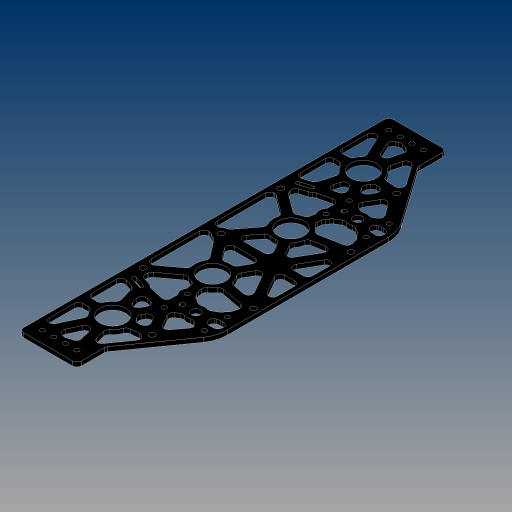
# Autodesk Inventor part: ELEV_027_GEARBOX1
Saved by Autodesk Inventor 2024.3 (Build 283343000, 343)
## iProperties
Created: 2024-12-02
Part Number: ELEV_027_GEARBOX1
Material: Aluminum 6061
Document SubType Name: Modeling
Designer: Kenji
Density: 2.7 g/cm^3
Appearance: Anodized - Black
Mass: 464.349 g
Surface Area: 813.217 cm^2
Volume: 171.981 cm^3
Author: Kenji
Autodesk Inventor part; units mm, degrees
(part 1 of 2)
ref_plane "YZ Plane" through (0, 0, 0) normal (1, 0, 0) x (0, 1, 0)
ref_plane "XZ Plane" through (0, 0, 0) normal (0, 1, 0) x (-1, 0, 0)
ref_plane "XY Plane" through (0, 0, 0) normal (0, 0, 1) x (1, 0, 0)
sketch "Sketch1" plane through (0, 0, 0) normal (0, 1, 0) x (-1, 0, 0)
  line L0 (0, 0) -> (63.5, 0) construction
  line L1 (63.5, 0) -> (63.5, -25.4) construction
  line L2 (63.5, -25.4) -> (0, -25.4) construction
  line L3 (0, -25.4) -> (0, 0) construction
  line L4 (0, -381) -> (63.5, -381) construction
  line L5 (63.5, -381) -> (63.5, -406.4) construction
  line L6 (63.5, -406.4) -> (0, -406.4) construction
  line L7 (0, -406.4) -> (0, -381) construction
  circle A0 centre (26.0346, -341.0966) radius 22.733 construction
  circle A1 centre (26.0346, -65.3034) radius 22.733 construction
  line L8 (26.0346, -65.3034) -> (26.0346, -341.0966) construction
  line L9 (63.5, -203.2) -> (-50.8, -203.2) construction
  circle A2 centre (26.0346, -65.3034) radius 14.2875
  circle A3 centre (26.0346, -341.0966) radius 14.2875
  circle A4 centre (26.0346, -65.3034) radius 27.2288 construction
  circle A5 centre (26.0346, -341.0966) radius 27.2288 construction
  circle A6 centre (692.1496, -341.0966) radius 22.733 construction
  circle A7 centre (692.1496, -341.0966) radius 27.2288 construction
  line L10 (-50.8, 0) -> (-50.8, -406.4) construction
  circle A8 centre (-16.5354, -292.1) radius 31.7246 construction
  circle A9 centre (-16.5354, -114.3) radius 31.7246 construction
  circle A10 centre (-16.5354, -292.1) radius 10.16 construction
  circle A11 centre (-16.5354, -114.3) radius 10.16 construction
  circle A12 centre (-16.5354, -292.1) radius 5
  circle A13 centre (-16.5354, -114.3) radius 5
  line L11 (692.1496, -363.8296) -> (26.0346, -363.8296) construction
  line L12 (-48.26, -114.3) -> (-50.8, -114.3) construction
  line L13 (63.5, -25.4) -> (63.5, -381) construction
  line L14 (-48.26, -292.1) -> (-50.8, -292.1) construction
  circle A14 centre (10.9389, -160.02) radius 43.18 construction
  circle A15 centre (10.9389, -160.02) radius 45.72 construction
  circle A16 centre (10.9389, -246.38) radius 43.18 construction
  line L15 (10.9389, -160.02) -> (10.9389, -246.38) construction
  circle A17 centre (10.9389, -160.02) radius 14.2875
  circle A18 centre (10.9389, -246.38) radius 14.2875
  circle A19 centre (10.9389, -246.38) radius 45.72 construction
  line L16 (10.9389, -203.2) -> (63.5, -203.2) construction
  circle A20 centre (10.9389, -160.02) radius 14.3256 construction
  circle A21 centre (26.0346, -65.3034) radius 28.6512 construction
  circle A22 centre (26.0346, -341.0966) radius 28.6512 construction
  circle A23 centre (10.9389, -246.38) radius 14.3256 construction
  line L17 (53.3378, -73.9883) -> (24.5905, -164.3625) construction
  line L18 (-2.6157, -65.0706) -> (-3.3862, -159.9036) construction
  line L19 (53.3378, -332.4117) -> (24.5905, -242.0375) construction
  line L20 (-3.3862, -246.4964) -> (-2.6157, -341.3294) construction
  circle A24 centre (12.7, -12.7) radius 2.54
  line L21 (63.5, -12.7) -> (0, -12.7) construction
  circle A25 centre (25.4, -12.7) radius 2.54
  circle A26 centre (38.1, -12.7) radius 2.54
  circle A27 centre (50.8, -12.7) radius 2.54
  circle A28 centre (12.7, -393.7) radius 2.54
  circle A29 centre (25.4, -393.7) radius 2.54
  circle A30 centre (38.1, -393.7) radius 2.54
  circle A31 centre (50.8, -393.7) radius 2.54
  line L22 (63.5, -401.6375) -> (63.5, -4.7625)
  line L23 (58.7375, 0) -> (4.7625, 0)
  line L24 (0, -4.7625) -> (0, -25.4)
  circle A32 centre (-16.5354, -114.3) radius 34.2646 construction
  line L25 (0, 0) -> (-50.8, 0) construction
  line L26 (-50.8, 0) -> (-50.8, -25.4) construction
  line L27 (-50.8, -25.4) -> (0, -25.4) construction
  line L28 (0, -25.4) -> (0, 0) construction
  line L29 (0, -25.4) -> (0, -30.2327)
  line L30 (-0.8777, -32.9877) -> (-44.4852, -94.479)
  arc A33 (-0.8777, -32.9877) -> (0, -30.2327) centre (-4.7625, -30.2327) ccw
  circle A34 centre (-16.5354, -292.1) radius 34.2646 construction
  line L31 (-50.8, -114.3) -> (-50.8, -292.1)
  line L32 (58.7375, -406.4) -> (4.7625, -406.4)
  line L33 (0, -381) -> (0, -401.6375)
  line L34 (0, -381) -> (0, -376.1673)
  line L35 (-0.8777, -373.4123) -> (-44.4852, -311.921)
  arc A35 (0, -376.1673) -> (-0.8777, -373.4123) centre (-4.7625, -376.1673) ccw
  arc A36 (-44.4852, -94.479) -> (-50.8, -114.3) centre (-16.5354, -114.3) ccw
  arc A37 (-50.8, -292.1) -> (-44.4852, -311.921) centre (-16.5354, -292.1) ccw
  arc A38 (4.7625, 0) -> (0, -4.7625) centre (4.7625, -4.7625) ccw
  arc A39 (63.5, -4.7625) -> (58.7375, 0) centre (58.7375, -4.7625) ccw
  arc A40 (58.7375, -406.4) -> (63.5, -401.6375) centre (58.7375, -401.6375) ccw
  arc A41 (0, -401.6375) -> (4.7625, -406.4) centre (4.7625, -401.6375) ccw
  circle A42 centre (50.2604, -112.9905) radius 6.35 construction
  circle A43 centre (50.2604, -112.9905) radius 3.175 construction
  line L36 (50.2604, -112.9905) -> (41.7887, -110.2957) construction
  circle A44 centre (50.2604, -112.9905) radius 1.9844 construction
  line L37 (50.2604, -112.9905) -> (38.1579, -109.1408) construction
  circle A45 centre (38.1579, -109.1408) radius 1.9844 construction
  line L38 (50.8619, -111.0995) -> (38.7594, -107.2498)
  line L39 (49.6589, -114.8815) -> (37.5564, -111.0318)
  arc A46 (49.6589, -114.8815) -> (50.8619, -111.0995) centre (50.2604, -112.9905) ccw
  arc A47 (38.7594, -107.2498) -> (37.5564, -111.0318) centre (38.1579, -109.1408) ccw
  line L40 (50.8619, -295.3005) -> (38.7594, -299.1502)
  line L41 (49.6589, -291.5185) -> (37.5564, -295.3682)
  arc A48 (50.8619, -295.3005) -> (49.6589, -291.5185) centre (50.2604, -293.4095) ccw
  arc A49 (37.5564, -295.3682) -> (38.7594, -299.1502) centre (38.1579, -297.2592) ccw
  circle A50 centre (44.3715, -203.2) radius 6.35 construction
  circle A51 centre (54.8316, -127.5288) radius 6.35 construction
  circle A52 centre (-13.904, -68.6812) radius 6.35 construction
  circle A53 centre (-44.45, -149.4985) radius 6.35 construction
  line L42 (-33.9779, -151.4878) -> (-38.2116, -150.6836) construction
  line L43 (-37.8265, -141.1468) -> (-40.5043, -144.5232) construction
  circle A54 centre (-44.45, -149.4985) radius 3.2512
  line L44 (-2.5147, -67.718) -> (-7.5766, -68.1461) construction
  line L45 (-14.2697, -75.0207) -> (-14.5622, -80.0923) construction
  circle A55 centre (-13.904, -68.6812) radius 3.2512
  line L46 (52.927, -121.4712) -> (52.1651, -119.0481) construction
  line L47 (49.7278, -131.3068) -> (47.6863, -132.8181) construction
  line L48 (40.484, -198.1791) -> (38.929, -196.1707) construction
  line L49 (40.484, -208.2209) -> (38.929, -210.2293) construction
  circle A56 centre (54.8316, -127.5288) radius 3.2512
  circle A57 centre (44.3715, -203.2) radius 3.2512
  circle A58 centre (54.8316, -278.8712) radius 6.35 construction
  circle A59 centre (-13.904, -337.7188) radius 6.35 construction
  circle A60 centre (-44.45, -256.9015) radius 6.35 construction
  circle A61 centre (-44.45, -256.9015) radius 3.2512
  circle A62 centre (-13.904, -337.7188) radius 3.2512
  circle A63 centre (54.8316, -278.8712) radius 3.2512
  circle A64 centre (-16.5354, -114.3) radius 25.4 construction
  circle A65 centre (-16.5354, -88.9) radius 2.54 construction
  circle A66 centre (-29.2354, -92.303) radius 2.54 construction
  circle A67 centre (-38.5324, -101.6) radius 2.54
  circle A68 centre (-41.9354, -114.3) radius 2.54 construction
  circle A69 centre (-38.5324, -127) radius 2.54
  circle A70 centre (-29.2354, -136.297) radius 2.54 construction
  circle A71 centre (-16.5354, -139.7) radius 2.54 construction
  circle A72 centre (-3.8354, -136.297) radius 2.54 construction
  circle A73 centre (5.4616, -127) radius 2.54
  circle A74 centre (8.8646, -114.3) radius 2.54 construction
  circle A75 centre (5.4616, -101.6) radius 2.54
  circle A76 centre (-3.8354, -92.303) radius 2.54 construction
  circle A77 centre (-16.5354, -317.5) radius 2.54 construction
  circle A78 centre (-38.5324, -304.8) radius 2.54
  circle A79 centre (-38.5324, -279.4) radius 2.54
  circle A80 centre (-16.5354, -266.7) radius 2.54 construction
  circle A81 centre (5.4616, -279.4) radius 2.54
  circle A82 centre (5.4616, -304.8) radius 2.54
  circle A83 centre (50.2604, -112.9905) radius 8.89 construction
  line L50 (26.0346, -341.0966) -> (54.8316, -278.8712) construction
  line L51 (26.0346, -341.0966) -> (-13.904, -337.7188) construction
  line L52 (26.0346, -341.0966) -> (12.7, -393.7) construction
  point P0 (0, -31.75)
  point P1 (0, -374.65)
  dimension "d18" = 63.4492
  dimension "d26" = 63.4492
  dimension "d77" = 12.7
  dimension "d93" = 50.8
  dimension "d0" = 25.4
  dimension "d1" = 63.5
  dimension "d2" = 406.4
  dimension "d3" = 45.466
  dimension "d4" = 65.3034
  dimension "d5" = 203.2
  dimension "d6" = 28.575
  dimension "d7" = 54.4576
  dimension "d13" = 692.1496
  dimension "d14" = 50.8
  dimension "d19" = 20.32
  dimension "d33" = 10
  dimension "d34" = 666.115
  dimension "d35" = 2.54
  dimension "d48" = 2.54
  dimension "d49" = 86.36
  dimension "d50" = 28.575
  dimension "d51" = 28.575
  dimension "d52" = 43.18
  dimension "d53" = 177.8
  dimension "d54" = 177.8
  dimension "d56" = 57.3024
  dimension "d58" = 28.6512
  dimension "d59" = 12.7
  dimension "d60" = 5.08
  dimension "d63" = 12.7
  dimension "d68" = 2.54
  dimension "d69" = 25.4
  dimension "d70" = 6.35
  dimension "d71" = 4.7625
  dimension "d72" = 2.54
  dimension "d73" = 6.35
  dimension "d74" = 4.7625
  dimension "d75" = 4.7625
  dimension "d76" = 4.7625
  dimension "d78" = 6.35
  dimension "d81" = 38.1
  dimension "d83" = 3.9688
  dimension "d84" = 12.7
  dimension "d85" = 12.7
  dimension "d86" = 6.5024
  dimension "d87" = 5.08
  dimension "d88" = 6.5024
  dimension "d89" = 2.54
  dimension "d90" = 6.5024
  dimension "d91" = 2.54
  dimension "d92" = 6.5024
  dimension "d94" = 5.08
  dimension "d97" = 360
  dimension "d102" = 2.54
  dimension "d207" = 68.5658
  dimension "d209" = 40.0812
  dimension "d211" = 54.2672
  dimension "d215" = 24.834
  dimension "d216" = 85.166
  dimension "d217" = 80.61
  constraints: 106 end point, 77 centre point, 54 point on circle, 40 point on line, 32 tangent, 26 coincident, 22 symmetric about line, 15 equal radius, 7 horizontal, 7 parallel, 7 perpendicular, 6 collinear, 6 equal length, 6 midpoint, 6 vertical, 4 vertical alignment, 3 concentric, 3 horizontal alignment, 68 other
  measures "d0" distance between parallel lines of L0 L2
  measures "d1" distance of L0.start L0.end
  measures "d2" distance between parallel lines of L6 L0
  measures "d3" diameter of A1
  measures "d4" distance from line of L6 L8.end
  measures "d5" distance between parallel lines of L6 L9
  measures "d6" diameter of A2
  measures "d7" diameter of A4
  measures "d13" distance from line of L7 point (692.15, -341.097)
  measures "d14" distance between parallel lines of L10 L7
  measures "d19" diameter of A10
  measures "d33" diameter of A13
  measures "d34" distance of L11.start L11.end
  measures "d35" distance of L12.start L12.end
  measures "d48" radial gap between concentric circles of A14 A15
  measures "d49" diameter of A14
  measures "d50" diameter of A17
  measures "d51" diameter of A18
  measures "d52" distance from line of L15.start L16
  measures "d53" distance between parallel lines of L4 L16
  measures "d54" distance of A34.centre A32.centre
  measures "d56" diameter of A21
  measures "d58" diameter of A20
  measures "d59" distance from line of L3 A24.centre
  measures "d60" diameter of A24
  measures "d63" distance of A24.centre A25.centre
  measures "d69" distance between parallel lines of L25 L27
  measures "d70" distance of L27.end point (0, -31.75)
  measures "d71" radius of A33
  measures "d73" distance of L4.start point (0, -374.65)
  measures "d74" radius of A35
  measures "d75" radius of A38
  measures "d76" radius of A39
  measures "d78" diameter of A43
  measures "d81" distance of L36.end L17.start
  measures "d83" diameter of A44
  measures "d84" distance of L37.start L37.end
  measures "d85" diameter of A50
  measures "d86" diameter of A54
  measures "d87" distance of L44.start L44.end
  measures "d88" diameter of A55
  measures "d89" distance of L46.start L46.end
  measures "d90" diameter of A56
  measures "d91" distance of L48.start L48.end
  measures "d92" diameter of A57
  measures "d94" diameter of A65
  measures "d207" distance of L50.start L50.end
  measures "d209" distance of L50.start A59.centre
  measures "d211" distance of L50.start L52.end
  measures "d215" angle of L8 L50
  measures "d216" angle of L51 L8
  measures "d217" angle of L51 L52
extrude "Extrusion1" add sketch "Sketch1" along normal blind 4.7625
sketch "Sketch2" plane through (0, 4.7625, 0) normal (0, 1, 0) x (1, 0, 0)
  line L0 (-63.5, 401.6375) -> (-63.5, 4.7625) construction
  arc A0 (-63.5, 4.7625) -> (-58.7375, 0) centre (-58.7375, 4.7625) ccw construction
  line L1 (-58.7375, 0) -> (-4.7625, 0) construction
  arc A1 (-4.7625, 0) -> (0, 4.7625) centre (-4.7625, 4.7625) ccw construction
  line L2 (0, 4.7625) -> (0, 30.2327) construction
  arc A2 (0.8777, 32.9877) -> (0, 30.2327) centre (4.7625, 30.2327) ccw construction
  line L3 (0.8777, 32.9877) -> (44.4852, 94.479) construction
  arc A3 (44.4852, 94.479) -> (50.8, 114.3) centre (16.5354, 114.3) ccw construction
  line L4 (50.8, 114.3) -> (50.8, 292.1) construction
  arc A4 (50.8, 292.1) -> (44.4852, 311.921) centre (16.5354, 292.1) ccw construction
  line L5 (44.4852, 311.921) -> (0.8777, 373.4123) construction
  arc A5 (0, 376.1673) -> (0.8777, 373.4123) centre (4.7625, 376.1673) ccw construction
  line L6 (0, 376.1673) -> (0, 401.6375) construction
  arc A6 (0, 401.6375) -> (-4.7625, 406.4) centre (-4.7625, 401.6375) ccw construction
  line L7 (-4.7625, 406.4) -> (-58.7375, 406.4) construction
  arc A7 (-58.7375, 406.4) -> (-63.5, 401.6375) centre (-58.7375, 401.6375) ccw construction
  circle A8 centre (38.5324, 304.8) radius 2.54 construction
  circle A9 centre (-5.4616, 304.8) radius 2.54 construction
  circle A10 centre (-5.4616, 127) radius 2.54 construction
  circle A11 centre (38.5324, 127) radius 2.54 construction
  circle A12 centre (44.45, 256.9015) radius 3.2512 construction
  circle A13 centre (-44.3715, 203.2) radius 3.2512 construction
  circle A14 centre (44.45, 149.4985) radius 3.2512 construction
  circle A15 centre (-25.4, 393.7) radius 2.54 construction
  circle A16 centre (-50.8, 393.7) radius 2.54 construction
  circle A17 centre (-38.1, 12.7) radius 2.54 construction
  circle A18 centre (-26.0346, 65.3034) radius 14.2875 construction
  circle A19 centre (-26.0346, 341.0966) radius 14.2875 construction
  circle A20 centre (16.5354, 292.1) radius 5 construction
  circle A21 centre (16.5354, 114.3) radius 5 construction
  circle A22 centre (-10.9389, 160.02) radius 14.2875 construction
  circle A23 centre (-10.9389, 246.38) radius 14.2875 construction
  circle A24 centre (-12.7, 12.7) radius 2.54 construction
  circle A25 centre (-25.4, 12.7) radius 2.54 construction
  circle A26 centre (-50.8, 12.7) radius 2.54 construction
  circle A27 centre (-38.1, 393.7) radius 2.54 construction
  circle A28 centre (-12.7, 393.7) radius 2.54 construction
  circle A29 centre (-54.8316, 127.5288) radius 3.2512 construction
  circle A30 centre (-54.8316, 278.8712) radius 3.2512 construction
  circle A31 centre (38.5324, 101.6) radius 2.54 construction
  circle A32 centre (-5.4616, 101.6) radius 2.54 construction
  circle A33 centre (-5.4616, 279.4) radius 2.54 construction
  circle A34 centre (38.5324, 279.4) radius 2.54 construction
  circle A35 centre (13.904, 337.7188) radius 3.2512 construction
  circle A36 centre (13.904, 68.6812) radius 3.2512 construction
  line L8 (-50.8619, 295.3005) -> (-38.7594, 299.1502) construction
  arc A37 (-37.5564, 295.3682) -> (-38.7594, 299.1502) centre (-38.1579, 297.2592) ccw construction
  line L9 (-37.5564, 295.3682) -> (-49.6589, 291.5185) construction
  arc A38 (-50.8619, 295.3005) -> (-49.6589, 291.5185) centre (-50.2604, 293.4095) ccw construction
  line L10 (-49.6589, 114.8815) -> (-37.5564, 111.0318) construction
  arc A39 (-38.7594, 107.2498) -> (-37.5564, 111.0318) centre (-38.1579, 109.1408) ccw construction
  line L11 (-38.7594, 107.2498) -> (-50.8619, 111.0995) construction
  arc A40 (-49.6589, 114.8815) -> (-50.8619, 111.0995) centre (-50.2604, 112.9905) ccw construction
  line L12 (-58.7375, 4.7625) -> (-58.7375, 401.6375) construction
  line L13 (-58.7375, 401.6375) -> (-4.7625, 401.6375) construction
  line L14 (-4.7625, 401.6375) -> (-4.7625, 376.1673) construction
  arc A41 (-4.7625, 376.1673) -> (-3.0071, 370.6574) centre (4.7625, 376.1673) ccw construction
  line L15 (-3.0071, 370.6574) -> (40.6004, 309.166) construction
  arc A42 (46.0375, 292.1) -> (40.6004, 309.166) centre (16.5354, 292.1) ccw construction
  line L16 (46.0375, 292.1) -> (46.0375, 203.2) construction
  circle A43 centre (-50.8, 393.7) radius 7.3025 construction
  circle A44 centre (-38.1, 393.7) radius 7.3025 construction
  circle A45 centre (-25.4, 393.7) radius 7.3025 construction
  circle A46 centre (-12.7, 393.7) radius 7.3025 construction
  circle A47 centre (-26.0346, 341.0966) radius 19.05 construction
  circle A48 centre (13.904, 337.7188) radius 8.0137 construction
  circle A49 centre (-5.4616, 304.8) radius 7.3025 construction
  circle A50 centre (-5.4616, 279.4) radius 7.3025 construction
  circle A51 centre (-10.9389, 246.38) radius 19.05 construction
  line L17 (-48.2152, 286.98) -> (-36.1128, 290.8297) construction
  arc A52 (-36.1128, 290.8297) -> (-40.2031, 303.6886) centre (-38.1579, 297.2592) ccw construction
  line L18 (-40.2031, 303.6886) -> (-52.3056, 299.8389) construction
  arc A53 (-52.3056, 299.8389) -> (-48.2152, 286.98) centre (-50.2604, 293.4095) ccw construction
  circle A54 centre (-54.8316, 278.8712) radius 8.0137 construction
  circle A55 centre (-44.3715, 203.2) radius 8.0137 construction
  circle A56 centre (16.5354, 292.1) radius 9.7625 construction
  circle A57 centre (38.5324, 279.4) radius 7.3025 construction
  circle A58 centre (44.45, 256.9015) radius 8.0137 construction
  circle A59 centre (38.5324, 304.8) radius 7.3025 construction
  line L19 (-58.7375, 203.2) -> (46.0375, 203.2) construction
  line L20 (-39.4655, 209.5364) -> (-22.6014, 231.3172) construction
  line L21 (-26.2503, 257.7141) -> (-48.3906, 274.1033) construction
  line L22 (-31.5836, 298.7754) -> (-12.5774, 303.1589) construction
  line L23 (-7.8215, 265.1732) -> (-6.6566, 272.1959) construction
  line L24 (7.7764, 249.9351) -> (36.5771, 255.406) construction
  line L25 (42.4116, 264.6516) -> (40.39, 272.3377) construction
  line L26 (24.99, 287.2188) -> (32.2083, 283.0513) construction
  line L27 (0.8625, 283.0513) -> (8.0808, 287.2188) construction
  line L28 (0.8625, 301.1488) -> (8.0808, 296.9813) construction
  line L29 (24.99, 296.9813) -> (32.2083, 301.1488) construction
  line L30 (18.7047, 331.3021) -> (34.1578, 310.6472) construction
  line L31 (-9.0625, 311.153) -> (-16.641, 324.5236) construction
  line L32 (-1.7589, 311.0941) -> (9.8407, 330.8116) construction
  line L33 (-7.0523, 339.4912) -> (5.9188, 338.3941) construction
  line L34 (-21.3536, 359.5625) -> (-14.4944, 386.6214) construction
  line L35 (-34.1489, 358.332) -> (-47.6895, 387.0931) construction
  line L36 (-36.3596, 303.762) -> (-31.1123, 322.7358) construction
  line L37 (-54.8316, 278.8712) -> (-50.2604, 293.4095) construction
  line L38 (-5.4616, 286.7025) -> (-5.4616, 297.4975) construction
  line L39 (40.4726, 249.9445) -> (13.7479, 203.2) construction
  line L40 (-1.4838, 229.842) -> (13.7479, 203.2) construction
  line L41 (-45.0846, 341.0966) -> (-58.7375, 341.0966) construction
  line L42 (-47.8591, 345.8591) -> (-53.975, 345.8591)
  line L43 (-50.8, 393.7) -> (-58.7375, 393.7) construction
  line L44 (-39.6396, 358.8137) -> (-49.6661, 380.1107)
  arc A60 (-40.3657, 353.6474) -> (-43.4942, 348.7166) centre (-26.0346, 341.0966) ccw
  line L45 (-58.7375, 350.6216) -> (-58.7375, 378.0821)
  arc A61 (-47.8591, 345.8591) -> (-43.4942, 348.7166) centre (-47.8591, 350.6216) ccw
  arc A62 (-40.3657, 353.6474) -> (-39.6396, 358.8137) centre (-43.9484, 356.7851) ccw
  arc A63 (-58.7375, 350.6216) -> (-53.975, 345.8591) centre (-53.975, 350.6216) ccw
  arc A64 (-49.6661, 380.1107) -> (-58.7375, 378.0821) centre (-53.975, 378.0821) ccw
  line L46 (-33.046, 367.1702) -> (-39.1165, 380.0643)
  line L47 (-24.1207, 368.0285) -> (-20.9678, 380.4662)
  arc A65 (-36.1072, 386.6747) -> (-34.2566, 387.4908) centre (-38.1, 393.7) ccw
  arc A66 (-29.2434, 387.4908) -> (-25.5116, 386.3984) centre (-25.4, 393.7) ccw
  arc A67 (-33.046, 367.1702) -> (-24.1207, 368.0285) centre (-28.7371, 369.1988) ccw
  arc A68 (-36.1072, 386.6747) -> (-39.1165, 380.0643) centre (-34.8076, 382.0929) ccw
  arc A69 (-29.2434, 387.4908) -> (-34.2566, 387.4908) centre (-31.75, 383.4413) ccw
  circle A70 centre (-25.5843, 381.6364) radius 4.7625 construction
  arc A71 (-20.9678, 380.4662) -> (-25.5116, 386.3984) centre (-25.5843, 381.6364) ccw
  line L48 (-16.0554, 361.0817) -> (-13.3658, 371.6918)
  line L49 (-3.8863, 344.0029) -> (5.8207, 343.1819)
  line L50 (-12.7, 393.7) -> (-4.7625, 393.7) construction
  line L51 (10.8092, 351.1749) -> (-4.8645, 373.2765)
  arc A72 (-7.9949, 347.2181) -> (-14.358, 356.1485) centre (-26.0346, 341.0966) ccw
  arc A73 (9.5261, 344.431) -> (9.0856, 344.1221) centre (13.904, 337.7188) ccw
  arc A74 (-16.0554, 361.0817) -> (-14.358, 356.1485) centre (-11.4389, 359.9115) ccw
  arc A75 (-7.9949, 347.2181) -> (-3.8863, 344.0029) centre (-3.485, 348.7485) ccw
  arc A76 (5.8207, 343.1819) -> (9.0856, 344.1221) centre (6.222, 347.9275) ccw
  arc A77 (9.5261, 344.431) -> (10.8092, 351.1749) centre (6.9244, 348.42) ccw
  circle A78 centre (-8.7493, 370.5216) radius 4.7625 construction
  arc A79 (-4.8645, 373.2765) -> (-13.3658, 371.6918) centre (-8.7493, 370.5216) ccw
  line L52 (-4.6891, 334.5118) -> (-1.5787, 334.2487)
  line L53 (-1.2033, 321.431) -> (2.1248, 327.0883)
  line L54 (-9.4515, 321.4974) -> (-11.1297, 324.4583)
  arc A80 (-10.796, 329.6646) -> (-9.2793, 332.0323) centre (-26.0346, 341.0966) ccw
  arc A81 (-10.796, 329.6646) -> (-11.1297, 324.4583) centre (-6.9864, 326.8067) ccw
  arc A82 (-4.6891, 334.5118) -> (-9.2793, 332.0323) centre (-5.0904, 329.7662) ccw
  arc A83 (2.1248, 327.0883) -> (-1.5787, 334.2487) centre (-1.9801, 329.5032) ccw
  arc A84 (-9.4515, 321.4974) -> (-1.2033, 321.431) centre (-5.3082, 323.8458) ccw
  line L55 (-47.8591, 336.3341) -> (-53.975, 336.3341)
  line L56 (-40.7412, 305.7855) -> (-36.442, 321.3311)
  line L57 (-56.6898, 291.3643) -> (-58.7375, 290.713) construction
  line L58 (-58.7375, 304.3029) -> (-58.7375, 331.5716)
  arc A85 (-43.4942, 333.4766) -> (-38.0327, 326.2997) centre (-26.0346, 341.0966) ccw
  arc A86 (-52.3056, 299.8389) -> (-52.4379, 299.7953) centre (-50.2604, 293.4095) ccw
  line L59 (-52.3056, 299.8389) -> (-43.8878, 302.5165)
  arc A87 (-43.8878, 302.5165) -> (-40.7412, 305.7855) centre (-45.3314, 307.055) ccw
  arc A88 (-36.442, 321.3311) -> (-38.0327, 326.2997) centre (-41.0322, 322.6005) ccw
  arc A89 (-43.4942, 333.4766) -> (-47.8591, 336.3341) centre (-47.8591, 331.5716) ccw
  arc A90 (-53.975, 336.3341) -> (-58.7375, 331.5716) centre (-53.975, 331.5716) ccw
  circle A91 centre (-53.975, 304.3029) radius 4.7625 construction
  arc A92 (-58.7375, 304.3029) -> (-52.4379, 299.7953) centre (-53.975, 304.3029) ccw
  line L60 (-29.3048, 311.4041) -> (-27.5732, 317.6656)
  line L61 (-23.6444, 305.494) -> (-18.9742, 306.5711)
  line L62 (-15.9012, 313.5602) -> (-18.8398, 318.7446)
  arc A93 (-26.3609, 322.0494) -> (-21.0825, 322.7015) centre (-26.0346, 341.0966) ccw
  arc A94 (-29.3048, 311.4041) -> (-23.6444, 305.494) centre (-24.7146, 310.1347) ccw
  arc A95 (-18.9742, 306.5711) -> (-15.9012, 313.5602) centre (-20.0445, 311.2118) ccw
  arc A96 (-18.8398, 318.7446) -> (-27.5732, 317.6656) centre (-22.983, 316.3962) ccw
  line L63 (-25.6468, 263.1927) -> (-45.1542, 277.6329)
  line L64 (-30.7922, 294.0704) -> (-16.0569, 297.4689)
  line L65 (-10.2241, 286.8053) -> (-10.2241, 292.8282)
  line L66 (-12.0658, 268.6897) -> (-11.3718, 272.8739)
  arc A97 (-15.5991, 264.8512) -> (-20.4384, 262.8925) centre (-10.9389, 246.38) ccw
  arc A98 (-11.2268, 283.8822) -> (-11.8825, 275.9217) centre (-5.4616, 279.4) ccw
  arc A99 (-46.9843, 280.4955) -> (-47.3989, 281.8669) centre (-54.8316, 278.8712) ccw
  arc A100 (-36.1128, 290.8297) -> (-33.2127, 292.6695) centre (-38.1579, 297.2592) ccw
  line L67 (-44.4253, 288.1856) -> (-36.1128, 290.8297)
  arc A101 (-25.6468, 263.1927) -> (-20.4384, 262.8925) centre (-22.8133, 267.0206) ccw
  arc A102 (-15.5991, 264.8512) -> (-12.0658, 268.6897) centre (-16.7641, 269.469) ccw
  arc A103 (-11.3718, 272.8739) -> (-11.8825, 275.9217) centre (-16.0701, 273.6532) ccw
  arc A104 (-11.2268, 283.8822) -> (-10.2241, 286.8053) centre (-14.9866, 286.8053) ccw
  arc A105 (-10.2241, 292.8282) -> (-16.0569, 297.4689) centre (-14.9866, 292.8282) ccw
  arc A106 (-30.7922, 294.0704) -> (-33.2127, 292.6695) centre (-29.7219, 289.4297) ccw
  arc A107 (-46.9843, 280.4955) -> (-45.1542, 277.6329) centre (-42.3206, 281.4608) ccw
  circle A108 centre (-42.9817, 283.6472) radius 4.7625 construction
  arc A109 (-44.4253, 288.1856) -> (-47.3989, 281.8669) centre (-42.9817, 283.6472) ccw
  line L68 (3.5125, 310.6622) -> (10.7493, 322.9636)
  line L69 (5.2361, 304.1229) -> (9.4199, 301.7074)
  line L70 (23.6509, 301.7074) -> (26.8599, 303.5601)
  line L71 (18.6675, 323.4018) -> (28.292, 310.5375)
  arc A110 (19.7173, 301.3294) -> (13.3535, 301.3294) centre (16.5354, 292.1) ccw
  arc A111 (1.7137, 306.1565) -> (1.4502, 307.1565) centre (-5.4616, 304.8) ccw
  arc A112 (3.5125, 310.6622) -> (5.2361, 304.1229) centre (7.6174, 308.2474) ccw
  arc A113 (9.4199, 301.7074) -> (13.3535, 301.3294) centre (11.8012, 305.8318) ccw
  arc A114 (19.7173, 301.3294) -> (23.6509, 301.7074) centre (21.2696, 305.8318) ccw
  arc A115 (26.8599, 303.5601) -> (28.292, 310.5375) centre (24.4786, 307.6845) ccw
  arc A116 (18.6675, 323.4018) -> (10.7493, 322.9636) centre (14.8541, 320.5488) ccw
  line L72 (38.5324, 279.4) -> (46.0375, 279.4) construction
  line L73 (33.2042, 287.9756) -> (34.5005, 287.2271)
  line L74 (33.2042, 296.2244) -> (34.5005, 296.9729)
  arc A117 (33.2042, 296.2244) -> (33.2042, 287.9756) centre (35.5854, 292.1) ccw
  arc A118 (40.1924, 286.5113) -> (37.5333, 286.6338) centre (38.5324, 279.4) ccw
  line L75 (46.0375, 291.1492) -> (46.0375, 292.1)
  arc A119 (37.5333, 297.5662) -> (39.6449, 297.5827) centre (38.5324, 304.8) ccw
  arc A120 (34.5005, 287.2271) -> (37.5333, 286.6338) centre (36.8818, 291.3515) ccw
  arc A121 (37.5333, 297.5662) -> (34.5005, 296.9729) centre (36.8818, 292.8485) ccw
  circle A122 centre (41.275, 291.1492) radius 4.7625 construction
  arc A123 (46.0375, 292.1) -> (39.6449, 297.5827) centre (40.49, 292.1) ccw
  arc A124 (40.1924, 286.5113) -> (46.0375, 291.1492) centre (41.275, 291.1492) ccw
  line L76 (-2.6692, 267.131) -> (-1.9752, 271.3152)
  line L77 (3.3328, 278.9782) -> (9.4199, 282.4926)
  line L78 (23.6509, 282.4926) -> (29.738, 278.9782)
  line L79 (37.2468, 265.565) -> (35.8103, 271.0268)
  line L80 (9.6134, 255.1317) -> (33.5298, 259.6748)
  arc A125 (4.792, 257.1244) -> (-0.5645, 262.3573) centre (-10.9389, 246.38) ccw
  arc A126 (-0.5077, 274.0348) -> (1.3026, 276.6483) centre (-5.4616, 279.4) ccw
  arc A127 (13.3535, 282.8706) -> (19.7173, 282.8706) centre (16.5354, 292.1) ccw
  arc A128 (31.7682, 276.6483) -> (34.0971, 273.5988) centre (38.5324, 279.4) ccw
  arc A129 (38.2047, 261.923) -> (37.2295, 260.3775) centre (44.45, 256.9015) ccw
  arc A130 (-2.6692, 267.131) -> (-0.5645, 262.3573) centre (2.0291, 266.3516) ccw
  arc A131 (4.792, 257.1244) -> (9.6134, 255.1317) centre (8.7247, 259.8105) ccw
  arc A132 (-0.5077, 274.0348) -> (-1.9752, 271.3152) centre (2.7231, 270.5358) ccw
  arc A133 (3.3328, 278.9782) -> (1.3026, 276.6483) centre (5.714, 274.8538) ccw
  arc A134 (13.3535, 282.8706) -> (9.4199, 282.4926) centre (11.8012, 278.3682) ccw
  arc A135 (23.6509, 282.4926) -> (19.7173, 282.8706) centre (21.2696, 278.3682) ccw
  arc A136 (31.7682, 276.6483) -> (29.738, 278.9782) centre (27.3568, 274.8538) ccw
  arc A137 (35.8103, 271.0268) -> (34.0971, 273.5988) centre (31.2044, 269.8154) ccw
  arc A138 (33.5298, 259.6748) -> (37.2468, 265.565) centre (32.641, 264.3536) ccw
  line L81 (-0.6991, 291.7403) -> (-0.6991, 292.4597)
  line L82 (2.8442, 294.5054) -> (3.4671, 294.1457)
  line L83 (2.8442, 289.6946) -> (3.4671, 290.0543)
  arc A139 (-0.6991, 291.7403) -> (2.8442, 289.6946) centre (1.6631, 291.7403) ccw
  arc A140 (2.8442, 294.5054) -> (-0.6991, 292.4597) centre (1.6631, 292.4597) ccw
  arc A141 (3.4671, 290.0543) -> (3.4671, 294.1457) centre (2.286, 292.1) ccw
  line L84 (-53.975, 207.9625) -> (-52.8865, 207.9625)
  line L85 (-58.7375, 212.725) -> (-58.7375, 266.1238)
  line L86 (-42.9243, 212.8484) -> (-28.0657, 232.039)
  line L87 (-31.3139, 255.537) -> (-50.8212, 269.9772)
  arc A142 (-45.8257, 211.0807) -> (-49.7125, 209.1744) centre (-44.3715, 203.2) ccw
  arc A143 (-29.5057, 250.6433) -> (-27.6529, 237.2397) centre (-10.9389, 246.38) ccw
  arc A144 (-54.2943, 270.8755) -> (-54.0935, 270.8916) centre (-54.8316, 278.8712) ccw
  arc A145 (-58.7375, 212.725) -> (-53.975, 207.9625) centre (-53.975, 212.725) ccw
  arc A146 (-52.8865, 207.9625) -> (-49.7125, 209.1744) centre (-52.8865, 212.725) ccw
  arc A147 (-45.8257, 211.0807) -> (-42.9243, 212.8484) centre (-46.69, 215.7641) ccw
  arc A148 (-28.0657, 232.039) -> (-27.6529, 237.2397) centre (-31.8314, 234.9547) ccw
  arc A149 (-29.5057, 250.6433) -> (-31.3139, 255.537) centre (-34.1474, 251.7092) ccw
  arc A150 (-50.8212, 269.9772) -> (-54.0935, 270.8916) centre (-53.6548, 266.1493) ccw
  arc A151 (-54.2943, 270.8755) -> (-58.7375, 266.1238) centre (-53.975, 266.1238) ccw
  line L88 (-28.716, 215.6406) -> (-20.5343, 226.2078)
  line L89 (-24.9504, 207.9625) -> (-2.6695, 207.9625)
  line L90 (-4.2413, 225.0696) -> (1.465, 215.0888)
  arc A152 (-2.6695, 207.9625) -> (1.465, 215.0888) centre (-2.6695, 212.725) ccw
  arc A153 (-28.716, 215.6406) -> (-24.9504, 207.9625) centre (-24.9504, 212.725) ccw
  arc A154 (-15.6027, 227.9097) -> (-8.8884, 227.4407) centre (-10.9389, 246.38) ccw
  arc A155 (-15.6027, 227.9097) -> (-20.5343, 226.2078) centre (-16.7686, 223.2921) ccw
  arc A156 (-4.2413, 225.0696) -> (-8.8884, 227.4407) centre (-8.3758, 222.7058) ccw
  line L91 (4.0277, 229.7971) -> (9.6134, 220.0272)
  line L92 (11.391, 245.774) -> (25.0344, 248.3657)
  line L93 (30.0577, 241.3231) -> (17.8824, 220.0272)
  arc A157 (4.342, 235.0047) -> (7.636, 242.1522) centre (-10.9389, 246.38) ccw
  arc A158 (9.6134, 220.0272) -> (17.8824, 220.0272) centre (13.7479, 222.3909) ccw
  arc A159 (30.0577, 241.3231) -> (25.0344, 248.3657) centre (25.9232, 243.6869) ccw
  arc A160 (11.391, 245.774) -> (7.636, 242.1522) centre (12.2798, 241.0952) ccw
  arc A161 (4.342, 235.0047) -> (4.0277, 229.7971) centre (8.1622, 232.1609) ccw
  line L94 (37.1405, 234.5209) -> (26.0308, 215.0888)
  line L95 (30.1653, 207.9625) -> (41.275, 207.9625)
  line L96 (46.0375, 212.725) -> (46.0375, 232.1571)
  arc A162 (46.0375, 232.1571) -> (37.1405, 234.5209) centre (41.275, 232.1571) ccw
  arc A163 (26.0308, 215.0888) -> (30.1653, 207.9625) centre (30.1653, 212.725) ccw
  arc A164 (41.275, 207.9625) -> (46.0375, 212.725) centre (41.275, 212.725) ccw
  line L97 (46.0375, 114.3) -> (46.0375, 203.2) construction
  circle A165 centre (-10.9389, 160.02) radius 19.05 construction
  line L98 (-48.2152, 119.42) -> (-36.1128, 115.5703) construction
  arc A166 (-40.2031, 102.7114) -> (-36.1128, 115.5703) centre (-38.1579, 109.1408) ccw construction
  circle A167 centre (-54.8316, 127.5288) radius 8.0137 construction
  circle A168 centre (-44.3715, 203.2) radius 8.0137 construction
  circle A169 centre (16.5354, 114.3) radius 9.7625 construction
  circle A170 centre (38.5324, 127) radius 7.3025 construction
  circle A171 centre (38.5324, 101.6) radius 7.3025 construction
  line L99 (-25.6468, 143.2073) -> (-45.1542, 128.7671)
  line L100 (-30.7922, 112.3296) -> (-16.0569, 108.9311)
  line L101 (-10.2241, 119.5947) -> (-10.2241, 113.5718)
  line L102 (-12.0658, 137.7103) -> (-11.3718, 133.5261)
  arc A172 (-20.4384, 143.5075) -> (-15.5991, 141.5488) centre (-10.9389, 160.02) ccw
  arc A173 (-11.8825, 130.4783) -> (-11.2268, 122.5178) centre (-5.4616, 127) ccw
  arc A174 (-47.3989, 124.5331) -> (-46.9843, 125.9045) centre (-54.8316, 127.5288) ccw
  arc A175 (-33.2127, 113.7305) -> (-36.1128, 115.5703) centre (-38.1579, 109.1408) ccw
  line L103 (-44.4253, 118.2144) -> (-36.1128, 115.5703)
  arc A176 (-20.4384, 143.5075) -> (-25.6468, 143.2073) centre (-22.8133, 139.3794) ccw
  arc A177 (-12.0658, 137.7103) -> (-15.5991, 141.5488) centre (-16.7641, 136.931) ccw
  arc A178 (-11.8825, 130.4783) -> (-11.3718, 133.5261) centre (-16.0701, 132.7468) ccw
  arc A179 (-10.2241, 119.5947) -> (-11.2268, 122.5178) centre (-14.9866, 119.5947) ccw
  arc A180 (-16.0569, 108.9311) -> (-10.2241, 113.5718) centre (-14.9866, 113.5718) ccw
  arc A181 (-33.2127, 113.7305) -> (-30.7922, 112.3296) centre (-29.7219, 116.9703) ccw
  arc A182 (-45.1542, 128.7671) -> (-46.9843, 125.9045) centre (-42.3206, 124.9392) ccw
  circle A183 centre (-42.9817, 122.7528) radius 4.7625 construction
  arc A184 (-47.3989, 124.5331) -> (-44.4253, 118.2144) centre (-42.9817, 122.7528) ccw
  line L104 (33.2042, 118.4244) -> (34.5005, 119.1729)
  line L105 (33.2042, 110.1756) -> (34.5005, 109.4271)
  arc A185 (33.2042, 118.4244) -> (33.2042, 110.1756) centre (35.5854, 114.3) ccw
  arc A186 (37.5333, 119.7662) -> (40.1924, 119.8887) centre (38.5324, 127) ccw
  line L106 (46.0375, 115.2508) -> (46.0375, 114.3)
  arc A187 (39.6449, 108.8173) -> (37.5333, 108.8338) centre (38.5324, 101.6) ccw
  arc A188 (37.5333, 119.7662) -> (34.5005, 119.1729) centre (36.8818, 115.0485) ccw
  arc A189 (34.5005, 109.4271) -> (37.5333, 108.8338) centre (36.8818, 113.5515) ccw
  arc A190 (39.6449, 108.8173) -> (46.0375, 114.3) centre (40.49, 114.3) ccw
  arc A191 (46.0375, 115.2508) -> (40.1924, 119.8887) centre (41.275, 115.2508) ccw
  line L107 (-2.6692, 139.269) -> (-1.9752, 135.0848)
  line L108 (3.3328, 127.4218) -> (9.4199, 123.9074)
  line L109 (23.6509, 123.9074) -> (29.738, 127.4218)
  line L110 (37.2468, 140.835) -> (35.8103, 135.3732)
  line L111 (9.6134, 151.2683) -> (33.5298, 146.7252)
  arc A192 (-0.5645, 144.0427) -> (4.792, 149.2756) centre (-10.9389, 160.02) ccw
  arc A193 (1.3026, 129.7517) -> (-0.5077, 132.3652) centre (-5.4616, 127) ccw
  arc A194 (19.7173, 123.5294) -> (13.3535, 123.5294) centre (16.5354, 114.3) ccw
  arc A195 (34.0971, 132.8012) -> (31.7682, 129.7517) centre (38.5324, 127) ccw
  arc A196 (-0.5645, 144.0427) -> (-2.6692, 139.269) centre (2.0291, 140.0484) ccw
  arc A197 (9.6134, 151.2683) -> (4.792, 149.2756) centre (8.7247, 146.5895) ccw
  arc A198 (-1.9752, 135.0848) -> (-0.5077, 132.3652) centre (2.7231, 135.8642) ccw
  arc A199 (1.3026, 129.7517) -> (3.3328, 127.4218) centre (5.714, 131.5462) ccw
  arc A200 (9.4199, 123.9074) -> (13.3535, 123.5294) centre (11.8012, 128.0318) ccw
  arc A201 (19.7173, 123.5294) -> (23.6509, 123.9074) centre (21.2696, 128.0318) ccw
  arc A202 (29.738, 127.4218) -> (31.7682, 129.7517) centre (27.3568, 131.5462) ccw
  arc A203 (34.0971, 132.8012) -> (35.8103, 135.3732) centre (31.2044, 136.5846) ccw
  arc A204 (37.2468, 140.835) -> (33.5298, 146.7252) centre (32.641, 142.0464) ccw
  line L112 (-53.975, 198.4375) -> (-52.8865, 198.4375)
  line L113 (-58.7375, 193.675) -> (-58.7375, 140.2762)
  line L114 (-42.9243, 193.5516) -> (-28.0657, 174.361)
  line L115 (-31.3139, 150.863) -> (-50.8212, 136.4228)
  arc A205 (-49.7125, 197.2256) -> (-45.8257, 195.3193) centre (-44.3715, 203.2) ccw
  arc A206 (-27.6529, 169.1603) -> (-29.5057, 155.7567) centre (-10.9389, 160.02) ccw
  arc A207 (-54.0935, 135.5084) -> (-54.2943, 135.5245) centre (-54.8316, 127.5288) ccw
  arc A208 (-53.975, 198.4375) -> (-58.7375, 193.675) centre (-53.975, 193.675) ccw
  arc A209 (-49.7125, 197.2256) -> (-52.8865, 198.4375) centre (-52.8865, 193.675) ccw
  arc A210 (-42.9243, 193.5516) -> (-45.8257, 195.3193) centre (-46.69, 190.6359) ccw
  arc A211 (-27.6529, 169.1603) -> (-28.0657, 174.361) centre (-31.8314, 171.4453) ccw
  arc A212 (-31.3139, 150.863) -> (-29.5057, 155.7567) centre (-34.1474, 154.6908) ccw
  arc A213 (-54.0935, 135.5084) -> (-50.8212, 136.4228) centre (-53.6548, 140.2507) ccw
  arc A214 (-58.7375, 140.2762) -> (-54.2943, 135.5245) centre (-53.975, 140.2762) ccw
  line L116 (-28.716, 190.7594) -> (-20.5343, 180.1922)
  line L117 (-24.9504, 198.4375) -> (-2.6695, 198.4375)
  line L118 (-4.2413, 181.3304) -> (1.465, 191.3112)
  arc A215 (1.465, 191.3112) -> (-2.6695, 198.4375) centre (-2.6695, 193.675) ccw
  arc A216 (-24.9504, 198.4375) -> (-28.716, 190.7594) centre (-24.9504, 193.675) ccw
  arc A217 (-8.8884, 178.9593) -> (-15.6027, 178.4903) centre (-10.9389, 160.02) ccw
  arc A218 (-20.5343, 180.1922) -> (-15.6027, 178.4903) centre (-16.7686, 183.1079) ccw
  arc A219 (-8.8884, 178.9593) -> (-4.2413, 181.3304) centre (-8.3758, 183.6942) ccw
  line L119 (4.0277, 176.6029) -> (9.6134, 186.3728)
  line L120 (11.391, 160.626) -> (25.0344, 158.0343)
  line L121 (30.0577, 165.0769) -> (17.8824, 186.3728)
  arc A220 (7.636, 164.2478) -> (4.342, 171.3953) centre (-10.9389, 160.02) ccw
  arc A221 (17.8824, 186.3728) -> (9.6134, 186.3728) centre (13.7479, 184.0091) ccw
  arc A222 (25.0344, 158.0343) -> (30.0577, 165.0769) centre (25.9232, 162.7131) ccw
  arc A223 (7.636, 164.2478) -> (11.391, 160.626) centre (12.2798, 165.3048) ccw
  arc A224 (4.0277, 176.6029) -> (4.342, 171.3953) centre (8.1622, 174.2391) ccw
  line L122 (37.1405, 171.8791) -> (26.0308, 191.3112)
  line L123 (30.1653, 198.4375) -> (41.275, 198.4375)
  line L124 (46.0375, 193.675) -> (46.0375, 174.2429)
  arc A225 (37.1405, 171.8791) -> (46.0375, 174.2429) centre (41.275, 174.2429) ccw
  arc A226 (30.1653, 198.4375) -> (26.0308, 191.3112) centre (30.1653, 193.675) ccw
  arc A227 (46.0375, 193.675) -> (41.275, 198.4375) centre (41.275, 193.675) ccw
  line L125 (-58.7375, 401.6375) -> (-58.7375, 4.7625) construction
  circle A228 centre (-25.4, 12.7) radius 7.3025 construction
  circle A229 centre (-26.0346, 65.3034) radius 19.05 construction
  circle A230 centre (13.904, 68.6812) radius 8.0137 construction
  line L126 (-40.2031, 102.7114) -> (-52.3056, 106.5611) construction
  circle A231 centre (16.5354, 114.3) radius 9.7625 construction
  line L127 (-47.8591, 60.5409) -> (-53.975, 60.5409)
  line L128 (-39.6396, 47.5863) -> (-49.6661, 26.2893)
  arc A232 (-43.4942, 57.6834) -> (-40.3657, 52.7526) centre (-26.0346, 65.3034) ccw
  line L129 (-58.7375, 55.7784) -> (-58.7375, 28.3179)
  arc A233 (-43.4942, 57.6834) -> (-47.8591, 60.5409) centre (-47.8591, 55.7784) ccw
  arc A234 (-39.6396, 47.5863) -> (-40.3657, 52.7526) centre (-43.9484, 49.6149) ccw
  arc A235 (-53.975, 60.5409) -> (-58.7375, 55.7784) centre (-53.975, 55.7784) ccw
  arc A236 (-58.7375, 28.3179) -> (-49.6661, 26.2893) centre (-53.975, 28.3179) ccw
  line L130 (-33.046, 39.2298) -> (-39.1165, 26.3357)
  line L131 (-24.1207, 38.3715) -> (-20.9678, 25.9338)
  arc A237 (-34.2566, 18.9092) -> (-36.1072, 19.7253) centre (-38.1, 12.7) ccw
  arc A238 (-25.5116, 20.0016) -> (-29.2434, 18.9092) centre (-25.4, 12.7) ccw
  arc A239 (-24.1207, 38.3715) -> (-33.046, 39.2298) centre (-28.7371, 37.2012) ccw
  arc A240 (-39.1165, 26.3357) -> (-36.1072, 19.7253) centre (-34.8076, 24.3071) ccw
  arc A241 (-34.2566, 18.9092) -> (-29.2434, 18.9092) centre (-31.75, 22.9587) ccw
  circle A242 centre (-25.5843, 24.7636) radius 4.7625 construction
  arc A243 (-25.5116, 20.0016) -> (-20.9678, 25.9338) centre (-25.5843, 24.7636) ccw
  line L132 (-16.0554, 45.3183) -> (-13.3658, 34.7082)
  line L133 (-3.8863, 62.3971) -> (5.8207, 63.2181)
  line L134 (10.8092, 55.2251) -> (-4.8645, 33.1235)
  arc A244 (-14.358, 50.2515) -> (-7.9949, 59.1819) centre (-26.0346, 65.3034) ccw
  arc A245 (9.0856, 62.2779) -> (9.5261, 61.969) centre (13.904, 68.6812) ccw
  arc A246 (-14.358, 50.2515) -> (-16.0554, 45.3183) centre (-11.4389, 46.4885) ccw
  arc A247 (-3.8863, 62.3971) -> (-7.9949, 59.1819) centre (-3.485, 57.6515) ccw
  arc A248 (9.0856, 62.2779) -> (5.8207, 63.2181) centre (6.222, 58.4725) ccw
  arc A249 (10.8092, 55.2251) -> (9.5261, 61.969) centre (6.9244, 57.98) ccw
  arc A250 (-13.3658, 34.7082) -> (-4.8645, 33.1235) centre (-8.7493, 35.8784) ccw
  line L135 (-4.6891, 71.8882) -> (-1.5787, 72.1513)
  line L136 (-1.2033, 84.969) -> (2.1248, 79.3117)
  line L137 (-9.4515, 84.9026) -> (-11.1297, 81.9417)
  arc A251 (-9.2793, 74.3677) -> (-10.796, 76.7354) centre (-26.0346, 65.3034) ccw
  arc A252 (-11.1297, 81.9417) -> (-10.796, 76.7354) centre (-6.9864, 79.5933) ccw
  arc A253 (-9.2793, 74.3677) -> (-4.6891, 71.8882) centre (-5.0904, 76.6338) ccw
  arc A254 (-1.5787, 72.1513) -> (2.1248, 79.3117) centre (-1.9801, 76.8968) ccw
  arc A255 (-1.2033, 84.969) -> (-9.4515, 84.9026) centre (-5.3082, 82.5542) ccw
  line L138 (-47.8591, 70.0659) -> (-53.975, 70.0659)
  line L139 (-40.7412, 100.6145) -> (-36.442, 85.0689)
  line L140 (-58.7375, 102.0971) -> (-58.7375, 74.8284)
  arc A256 (-38.0327, 80.1003) -> (-43.4942, 72.9234) centre (-26.0346, 65.3034) ccw
  line L141 (-52.3056, 106.5611) -> (-43.8878, 103.8835)
  arc A257 (-40.7412, 100.6145) -> (-43.8878, 103.8835) centre (-45.3314, 99.345) ccw
  arc A258 (-38.0327, 80.1003) -> (-36.442, 85.0689) centre (-41.0322, 83.7995) ccw
  arc A259 (-47.8591, 70.0659) -> (-43.4942, 72.9234) centre (-47.8591, 74.8284) ccw
  arc A260 (-58.7375, 74.8284) -> (-53.975, 70.0659) centre (-53.975, 74.8284) ccw
  circle A261 centre (-53.975, 102.0971) radius 4.7625 construction
  arc A262 (-52.4379, 106.6047) -> (-58.7375, 102.0971) centre (-53.975, 102.0971) ccw
  line L142 (-29.3048, 94.9959) -> (-27.5732, 88.7344)
  line L143 (-23.6444, 100.906) -> (-18.9742, 99.8289)
  line L144 (-15.9012, 92.8398) -> (-18.8398, 87.6554)
  arc A263 (-23.6444, 100.906) -> (-29.3048, 94.9959) centre (-24.7146, 96.2653) ccw
  arc A264 (-15.9012, 92.8398) -> (-18.9742, 99.8289) centre (-20.0445, 95.1882) ccw
  arc A265 (-27.5732, 88.7344) -> (-18.8398, 87.6554) centre (-22.983, 90.0038) ccw
  line L145 (3.5125, 95.7378) -> (10.7493, 83.4364)
  line L146 (5.2361, 102.2771) -> (9.4199, 104.6926)
  line L147 (23.6509, 104.6926) -> (26.8599, 102.8399)
  line L148 (18.6675, 82.9982) -> (28.292, 95.8625)
  arc A266 (13.3535, 105.0706) -> (19.7173, 105.0706) centre (16.5354, 114.3) ccw
  arc A267 (5.2361, 102.2771) -> (3.5125, 95.7378) centre (7.6174, 98.1526) ccw
  arc A268 (13.3535, 105.0706) -> (9.4199, 104.6926) centre (11.8012, 100.5682) ccw
  arc A269 (23.6509, 104.6926) -> (19.7173, 105.0706) centre (21.2696, 100.5682) ccw
  arc A270 (28.292, 95.8625) -> (26.8599, 102.8399) centre (24.4786, 98.7155) ccw
  arc A271 (10.7493, 83.4364) -> (18.6675, 82.9982) centre (14.8541, 85.8512) ccw
  line L149 (-0.6991, 114.6597) -> (-0.6991, 113.9403)
  line L150 (2.8442, 111.8946) -> (3.4671, 112.2543)
  line L151 (2.8442, 116.7054) -> (3.4671, 116.3457)
  arc A272 (2.8442, 116.7054) -> (-0.6991, 114.6597) centre (1.6631, 114.6597) ccw
  arc A273 (-0.6991, 113.9403) -> (2.8442, 111.8946) centre (1.6631, 113.9403) ccw
  arc A274 (3.4671, 112.2543) -> (3.4671, 116.3457) centre (2.286, 114.3) ccw
  line L152 (-58.7375, 401.6375) -> (-58.7375, 4.7625) construction
  arc A275 (-48.2152, 119.42) -> (-52.3056, 106.5611) centre (-50.2604, 112.9905) ccw construction
  line L153 (-40.7412, 100.6145) -> (-36.442, 85.0689)
  arc A276 (-52.4379, 106.6047) -> (-52.3056, 106.5611) centre (-50.2604, 112.9905) ccw
  line L154 (-52.3056, 106.5611) -> (-43.8878, 103.8835)
  arc A277 (-40.7412, 100.6145) -> (-43.8878, 103.8835) centre (-45.3314, 99.345) ccw
  circle A278 centre (-53.975, 102.0971) radius 4.7625 construction
  arc A279 (-52.4379, 106.6047) -> (-58.7375, 102.0971) centre (-53.975, 102.0971) ccw
  line L155 (-58.7375, 4.7625) -> (-58.7375, 401.6375) construction
  point P0 (-44.4797, 345.8591)
  point P1 (-58.7375, 345.8591)
  point P2 (-38.2001, 355.7561)
  point P3 (-52.7509, 386.6629)
  point P4 (-29.5824, 359.8133)
  point P5 (-42.9774, 388.2652)
  point P6 (-26.1187, 360.1464)
  point P7 (-16.8858, 357.8059)
  point P8 (-7.2538, 344.2877)
  point P9 (7.8833, 343.0075)
  point P10 (14.6966, 345.6932)
  point P11 (-8.0565, 334.7966)
  point P12 (-12.7961, 327.3983)
  point P13 (-44.4797, 336.3341)
  point P14 (-58.7375, 336.3341)
  point P15 (-41.429, 303.2987)
  point P16 (-35.5413, 324.5883)
  point P17 (-22.9306, 261.1821)
  point P18 (-46.818, 278.8645)
  point P19 (-32.4309, 293.6925)
  point P20 (-10.2241, 284.9358)
  point P21 (-12.6188, 265.3558)
  point P22 (-11.0658, 274.7182)
  point P23 (11.5364, 300.4855)
  point P24 (21.5344, 300.4855)
  point P25 (31.3571, 306.1565)
  point P26 (31.4028, 306.3796)
  point P27 (26.2969, 291.9634)
  point P28 (26.2969, 292.2366)
  point P29 (36.1196, 297.9077)
  point P30 (36.1196, 286.2923)
  point P31 (-3.2222, 263.7971)
  point P32 (-1.6692, 273.1595)
  point P33 (1.7137, 278.0435)
  point P34 (11.5364, 283.7145)
  point P35 (21.5344, 283.7145)
  point P36 (31.3571, 278.0435)
  point P37 (35.3347, 272.8349)
  point P38 (6.2934, 254.501)
  point P39 (-3.2222, 263.7971)
  point P40 (31.3571, 278.0435)
  point P41 (6.7739, 292.2366)
  point P42 (6.7739, 291.9634)
  point P43 (-58.7375, 207.9625)
  point P44 (-50.8165, 207.9625)
  point P45 (-58.7375, 271.8738)
  point P46 (-44.1915, 211.2117)
  point P47 (-25.9968, 234.7112)
  point P48 (-28.5977, 253.5264)
  point P49 (-52.485, 271.2088)
  point P50 (-18.4654, 228.8799)
  point P51 (-5.9186, 228.0034)
  point P52 (2.3504, 232.7309)
  point P53 (8.0709, 245.1434)
  point P54 (45.3857, 248.9426)
  point P55 (46.0375, 207.9625)
  point P56 (46.0375, 249.0466)
  point P57 (-11.0658, 131.6818)
  dimension "d103" = 4.7625
  dimension "d104" = 4.7625
  dimension "d105" = 4.7625
  dimension "d106" = 4.7625
  dimension "d107" = 4.7625
  dimension "d108" = 4.7625
  dimension "d109" = 4.7625
  dimension "d110" = 4.7625
  dimension "d111" = 4.7625
  dimension "d112" = 4.7625
  dimension "d113" = 4.7625
  dimension "d114" = 4.7625
  dimension "d115" = 4.7625
  dimension "d116" = 4.7625
  dimension "d117" = 4.7625
  dimension "d118" = 4.7625
  dimension "d119" = 4.7625
  dimension "d120" = 4.7625
  dimension "d122" = 4.7625
  dimension "d123" = 4.7625
  dimension "d124" = 4.7625
  dimension "d127" = 4.7625
  dimension "d128" = 4.7625
  dimension "d129" = 4.7625
  dimension "d130" = 4.7625
  dimension "d131" = 9.525
  dimension "d132" = 4.7625
  dimension "d133" = 4.7625
  dimension "d136" = 9.525
  dimension "d137" = 4.7625
  dimension "d138" = 9.525
  dimension "d139" = 4.7625
  dimension "d140" = 4.7625
  dimension "d141" = 4.7625
  dimension "d142" = 4.7625
  dimension "d143" = 4.7625
  dimension "d144" = 4.7625
  dimension "d146" = 4.7625
  dimension "d147" = 9.525
  dimension "d148" = 4.7625
  dimension "d149" = 4.7625
  dimension "d150" = 4.7625
  dimension "d151" = 4.7625
  dimension "d153" = 4.7625
  dimension "d154" = 4.7625
  dimension "d155" = 4.7625
  dimension "d156" = 4.7625
  dimension "d157" = 4.7625
  dimension "d158" = 4.7625
  dimension "d159" = 9.525
  dimension "d160" = 4.7625
  dimension "d161" = 4.7625
  dimension "d162" = 4.7625
  dimension "d163" = 4.7625
  dimension "d164" = 4.7625
  dimension "d170" = 4.7625
  dimension "d171" = 4.7625
  dimension "d172" = 4.7625
  dimension "d173" = 4.7625
  dimension "d174" = 9.525
  dimension "d175" = 4.7625
  dimension "d176" = 4.7625
  dimension "d177" = 4.7625
  dimension "d178" = 4.7625
  constraints: 494 point on circle, 288 end point, 270 symmetric about line, 226 centre point, 151 tangent, 127 point on line, 46 equal radius, 43 parallel, 12 concentric, 5 horizontal, 3 collinear, 3 vertical, 2 perpendicular, 263 other
  measures "d104" radial gap between concentric circles of A16 A43
  measures "d109" radial gap between concentric circles of A35 A48
  measures "d113" radial gap between concentric circles of A38 A53
  measures "d114" radial gap between concentric circles of A30 A54
  measures "d115" radial gap between concentric circles of A13 A55
  measures "d119" radial gap between concentric circles of A8 A59
  measures "d120" distance between parallel lines of L41 L42
  measures "d122" distance between parallel lines of L35 L44
  measures "d123" radius of A61
  measures "d124" radius of A63
  measures "d127" radius of A64
  measures "d128" distance between parallel lines of L35 L46
  measures "d129" distance between parallel lines of L34 L47
  measures "d130" radius of A67
  measures "d131" diameter of A70
  measures "d132" distance between parallel lines of L34 L48
  measures "d133" distance between parallel lines of L33 L49
  measures "d136" radius of A41
  measures "d137" radius of A74
  measures "d138" diameter of A78
  measures "d139" distance between parallel lines of L33 L52
  measures "d140" distance between parallel lines of L32 L53
  measures "d141" distance between parallel lines of L31 L54
  measures "d142" radius of A81